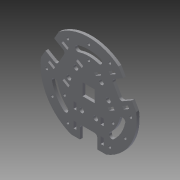
# Autodesk Inventor part: pcb
Saved by Autodesk Inventor 2015 (Build 190159000, 159)
## iProperties
Created: 2015-10-17
Part Number: pcb
Material: Polycarbonate, Clear
Document SubType Name: Modeling
Designer: Brian
Density: 1.2 g/cm^3
Appearance: Default
Mass: 22.2176 g
Surface Area: 156.183 cm^2
Volume: 18.5147 cm^3
Author: Brian
Autodesk Inventor part; units mm, degrees
ref_plane "YZ Plane" through (0, 0, 0) normal (1, 0, 0) x (0, 1, 0)
ref_plane "XZ Plane" through (0, 0, 0) normal (0, 1, 0) x (-1, 0, 0)
ref_plane "XY Plane" through (0, 0, 0) normal (0, 0, 1) x (1, 0, 0)
sketch "Sketch1" plane through (0, 0, 0) normal (0, 1, 0) x (-1, 0, 0)
  line L0 (0, 0) -> (0, -47.907) construction
  line L1 (0, -47.907) -> (18.8989, -47.907)
  line L2 (0, -47.907) -> (-18.8989, -47.907)
  line L3 (-41.4887, 23.9535) -> (0, 0) construction
  line L4 (0, 0) -> (41.4887, 23.9535) construction
  line L5 (41.4887, 23.9535) -> (32.0392, 40.3204)
  line L6 (-41.4887, 23.9535) -> (-50.9381, 7.5866)
  line L7 (-41.4887, 23.9535) -> (-32.0392, 40.3204)
  line L8 (41.4887, 23.9535) -> (50.9381, 7.5866)
  arc A0 (18.8989, -47.907) -> (50.9381, 7.5866) centre (0, 0) ccw
  arc A1 (32.0392, 40.3204) -> (-32.0392, 40.3204) centre (0, 0) ccw
  arc A2 (-50.9381, 7.5866) -> (-18.8989, -47.907) centre (0, 0) ccw
  dimension "d1" = 47.907
  dimension "d2" = 120
  dimension "d3" = 120
  dimension "d4" = 47.907
  dimension "d5" = 47.907
  dimension "d6" = 51.5
  dimension "d7" = 51.5
  dimension "d8" = 51.5
  constraints: 18 end point, 6 point on circle, 3 centre point, 3 perpendicular, 2 point on line, 1 coincident, 1 horizontal, 1 vertical
  measures "d1" distance of L0.start L0.end
  measures "d2" angle of L4 L0
  measures "d3" angle of L3 L4
  measures "d4" distance of L3.start L0.start
  measures "d5" distance of L0.start L4.end
  measures "d6" radius of A1
  measures "d7" radius of A2
  measures "d8" radius of A0
extrude "Extrusion1" add sketch "Sketch1" along normal blind 3
sketch "Sketch2" plane through (0, 3, 0) normal (0, 1, 0) x (1, 0, 0)
  circle A0 centre (-7.5, 20.006) radius 2.5
  circle A1 centre (7.5, 20.006) radius 2.5
  line L0 (-7.5, 20.006) -> (7.5, 20.006) construction
  point P0 (0, 0)
  point P1 (0, 20.006)
  dimension "d11" = 5
  dimension "d12" = 5
  dimension "d13" = 20.006
  dimension "d14" = 15
  constraints: 2 centre point, 2 end point, 1 horizontal, 1 horizontal alignment, 1 midpoint, 1 vertical alignment
  measures "d11" diameter of A0
  measures "d12" diameter of A1
  measures "d13" distance from line of point (0, 0) L0
  measures "d14" distance of L0.start L0.end
sketch "Sketch3" plane through (0, 3, 0) normal (0, 1, 0) x (1, 0, 0)
  line L0 (18.8989, 47.907) -> (-18.8989, 47.907) construction
  arc A0 (-18.8989, 47.907) -> (-50.9381, -7.5866) centre (0, 0) ccw construction
  line L1 (-50.9381, -7.5866) -> (-32.0392, -40.3204) construction
  arc A1 (-32.0392, -40.3204) -> (32.0392, -40.3204) centre (0, 0) ccw construction
  line L2 (32.0392, -40.3204) -> (50.9381, -7.5866) construction
  arc A2 (50.9381, -7.5866) -> (18.8989, 47.907) centre (0, 0) ccw construction
  line L3 (18.8989, 47.907) -> (-18.8989, 47.907)
  line L4 (18.8989, 47.907) -> (-18.8989, 47.907) projected
  line L5 (16, 40.907) -> (-16, 40.907) construction
  line L6 (16, 33.907) -> (-16, 33.907) construction
  line L7 (16, 22.907) -> (-16, 22.907) construction
  line L8 (16, 15.907) -> (-16, 15.907) construction
  line L9 (16, 15.907) -> (16, 40.907) construction
  line L10 (-16, 40.907) -> (-16, 15.907) construction
  line L11 (-16, 40.907) -> (-13, 40.907)
  line L12 (-13, 40.907) -> (-13, 33.907)
  line L13 (-13, 33.907) -> (-16, 33.907)
  line L14 (-16, 33.907) -> (-16, 40.907)
  line L15 (-16, 22.907) -> (-13, 22.907)
  line L16 (-13, 22.907) -> (-13, 15.907)
  line L17 (-13, 15.907) -> (-16, 15.907)
  line L18 (-16, 15.907) -> (-16, 22.907)
  line L19 (16, 15.907) -> (13, 15.907)
  line L20 (13, 15.907) -> (13, 22.907)
  line L21 (13, 22.907) -> (16, 22.907)
  line L22 (16, 22.907) -> (16, 15.907)
  line L23 (16, 33.907) -> (13, 33.907)
  line L24 (13, 33.907) -> (13, 40.907)
  line L25 (13, 40.907) -> (16, 40.907)
  line L26 (16, 40.907) -> (16, 33.907)
  point P0 (0, 15.907)
  dimension "d15" = 7
  dimension "d16" = 7
  dimension "d17" = 11
  dimension "d18" = 7
  dimension "d19" = 32
  dimension "d20" = 3
  dimension "d21" = 3
  constraints: 46 end point, 10 equal length, 10 point on line, 5 horizontal, 4 perpendicular, 1 midpoint, 1 vertical, 1 vertical alignment
  measures "d15" distance between parallel lines of L0 L5
  measures "d16" distance between parallel lines of L5 L6
  measures "d17" distance between parallel lines of L6 L7
  measures "d18" distance between parallel lines of L7 L8
  measures "d19" distance between parallel lines of L10 L9
  measures "d20" distance of L12.end L13.end
  measures "d21" distance of L24.end L25.end
extrude "Extrusion2" cut sketch "Sketch2" against normal blind 3
extrude "Extrusion3" cut sketch "Sketch3" against normal blind 3
sketch "Sketch4" plane through (0, 3, 0) normal (0, 1, 0) x (1, 0, 0)
  line L0 (-9.25, 33.907) -> (9.25, 33.907)
  line L1 (9.25, 33.907) -> (9.25, 47.907)
  line L2 (9.25, 47.907) -> (-9.25, 47.907)
  line L3 (-9.25, 47.907) -> (-9.25, 33.907)
  line L4 (18.8989, 47.907) -> (-18.8989, 47.907) projected
  point P0 (0, 0)
  point P1 (0, 33.907)
  dimension "d26" = 18.5
  dimension "d28" = 14
  constraints: 8 end point, 2 parallel, 1 horizontal, 1 midpoint, 1 perpendicular, 1 point on line, 1 vertical alignment
  measures "d26" distance of L0.start L0.end
  measures "d28" distance of L0.end L1.end
extrude "Extrusion4" cut sketch "Sketch4" against normal blind 3
sketch "Sketch5" plane through (0, 3, 0) normal (0, 1, 0) x (1, 0, 0)
  line L0 (-6.4, -6.4) -> (6.4, -6.4)
  line L1 (6.4, -6.4) -> (6.4, 6.4)
  line L2 (6.4, 6.4) -> (-6.4, 6.4)
  line L3 (-6.4, 6.4) -> (-6.4, -6.4)
  point P0 (0, 0)
  point P1 (0, 6.4)
  point P2 (-6.4, 0)
  dimension "d31" = 12.8
  dimension "d32" = 12.8
  constraints: 8 end point, 2 midpoint, 2 parallel, 1 horizontal, 1 horizontal alignment, 1 perpendicular, 1 vertical alignment
  measures "d31" distance of L0.end L1.end
  measures "d32" distance of L1.end L2.end
extrude "Extrusion5" cut sketch "Sketch5" against normal blind 3
pattern_circular "Circular Pattern1" count 3 over 360 about axis through (0, 0, 0) along (0, 1, 0) of "Extrusion4", "Extrusion2", "Extrusion3"
sketch "Sketch6" plane through (0, 3, 0) normal (0, 1, 0) x (1, 0, 0)
  line L0 (33.9893, -8.9428) -> (46.1137, -15.9428) construction
  line L1 (46.1137, -15.9428) -> (50.9381, -7.5866) construction
  arc A0 (50.9381, -7.5866) -> (18.8989, 47.907) centre (0, 0) ccw construction
  line L2 (18.8989, 47.907) -> (9.25, 47.907) construction
  line L3 (9.25, 47.907) -> (9.25, 33.907) construction
  line L4 (9.25, 33.907) -> (-9.25, 33.907) construction
  line L5 (-9.25, 33.907) -> (-9.25, 47.907) construction
  line L6 (-9.25, 47.907) -> (-18.8989, 47.907) construction
  arc A1 (-18.8989, 47.907) -> (-50.9381, -7.5866) centre (0, 0) ccw construction
  line L7 (-50.9381, -7.5866) -> (-46.1137, -15.9428) construction
  line L8 (-46.1137, -15.9428) -> (-33.9893, -8.9428) construction
  line L9 (-33.9893, -8.9428) -> (-24.7393, -24.9642) construction
  line L10 (-24.7393, -24.9642) -> (-36.8637, -31.9642) construction
  line L11 (-36.8637, -31.9642) -> (-32.0392, -40.3204) construction
  arc A2 (-32.0392, -40.3204) -> (32.0392, -40.3204) centre (0, 0) ccw construction
  line L12 (32.0392, -40.3204) -> (36.8637, -31.9642) construction
  line L13 (36.8637, -31.9642) -> (24.7393, -24.9642) construction
  line L14 (24.7393, -24.9642) -> (33.9893, -8.9428) construction
  line L15 (21.7759, 5.9029) -> (27.838, 2.4029) construction
  line L16 (27.838, 2.4029) -> (26.338, -0.1952) construction
  line L17 (26.338, -0.1952) -> (20.2759, 3.3048) construction
  line L18 (20.2759, 3.3048) -> (21.7759, 5.9029) construction
  line L19 (37.3643, -3.0971) -> (43.4265, -6.5971) construction
  line L20 (43.4265, -6.5971) -> (41.9265, -9.1952) construction
  line L21 (41.9265, -9.1952) -> (35.8643, -5.6952) construction
  line L22 (35.8643, -5.6952) -> (37.3643, -3.0971) construction
  line L23 (27.4265, -34.3099) -> (21.3643, -30.8099) construction
  line L24 (21.3643, -30.8099) -> (22.8643, -28.2118) construction
  line L25 (22.8643, -28.2118) -> (28.9265, -31.7118) construction
  line L26 (28.9265, -31.7118) -> (27.4265, -34.3099) construction
  line L27 (11.838, -25.3099) -> (5.7759, -21.8099) construction
  line L28 (5.7759, -21.8099) -> (7.2759, -19.2118) construction
  line L29 (7.2759, -19.2118) -> (13.338, -22.7118) construction
  line L30 (13.338, -22.7118) -> (11.838, -25.3099) construction
  circle A3 centre (21.0757, -3.5078) radius 2.5 construction
  circle A4 centre (13.5757, -16.4982) radius 2.5 construction
  line L31 (-5.7759, -21.8099) -> (-11.838, -25.3099) construction
  line L32 (-11.838, -25.3099) -> (-13.338, -22.7118) construction
  line L33 (-13.338, -22.7118) -> (-7.2759, -19.2118) construction
  line L34 (-7.2759, -19.2118) -> (-5.7759, -21.8099) construction
  line L35 (-21.3643, -30.8099) -> (-27.4265, -34.3099) construction
  line L36 (-27.4265, -34.3099) -> (-28.9265, -31.7118) construction
  line L37 (-28.9265, -31.7118) -> (-22.8643, -28.2118) construction
  line L38 (-22.8643, -28.2118) -> (-21.3643, -30.8099) construction
  line L39 (-43.4265, -6.5971) -> (-37.3643, -3.0971) construction
  line L40 (-37.3643, -3.0971) -> (-35.8643, -5.6952) construction
  line L41 (-35.8643, -5.6952) -> (-41.9265, -9.1952) construction
  line L42 (-41.9265, -9.1952) -> (-43.4265, -6.5971) construction
  line L43 (-27.838, 2.4029) -> (-21.7759, 5.9029) construction
  line L44 (-21.7759, 5.9029) -> (-20.2759, 3.3048) construction
  line L45 (-20.2759, 3.3048) -> (-26.338, -0.1952) construction
  line L46 (-26.338, -0.1952) -> (-27.838, 2.4029) construction
  circle A5 centre (-13.5757, -16.4982) radius 2.5 construction
  circle A6 centre (-21.0757, -3.5078) radius 2.5 construction
  line L47 (6.4, 6.4) -> (6.4, -6.4) construction
  line L48 (6.4, -6.4) -> (-6.4, -6.4) construction
  line L49 (-6.4, -6.4) -> (-6.4, 6.4) construction
  line L50 (-6.4, 6.4) -> (6.4, 6.4) construction
  line L51 (-16, 15.907) -> (-16, 22.907) construction
  line L52 (-16, 22.907) -> (-13, 22.907) construction
  line L53 (-13, 22.907) -> (-13, 15.907) construction
  line L54 (-13, 15.907) -> (-16, 15.907) construction
  line L55 (-16, 33.907) -> (-16, 40.907) construction
  line L56 (-16, 40.907) -> (-13, 40.907) construction
  line L57 (-13, 40.907) -> (-13, 33.907) construction
  line L58 (-13, 33.907) -> (-16, 33.907) construction
  line L59 (16, 40.907) -> (16, 33.907) construction
  line L60 (16, 33.907) -> (13, 33.907) construction
  line L61 (13, 33.907) -> (13, 40.907) construction
  line L62 (13, 40.907) -> (16, 40.907) construction
  line L63 (16, 22.907) -> (16, 15.907) construction
  line L64 (16, 15.907) -> (13, 15.907) construction
  line L65 (13, 15.907) -> (13, 22.907) construction
  line L66 (13, 22.907) -> (16, 22.907) construction
  circle A7 centre (-7.5, 20.006) radius 2.5 construction
  circle A8 centre (7.5, 20.006) radius 2.5 construction
  circle A9 centre (38.9711, 22.5) radius 1.5
  circle A10 centre (-38.9711, 22.5) radius 1.5
  circle A11 centre (0, -45) radius 1.5
  circle A12 centre (0, 0) radius 45 construction
  line L67 (0, 0) -> (38.9711, 22.5) construction
  line L68 (0, 0) -> (-38.9711, 22.5) construction
  circle A13 centre (0, 0) radius 30 construction
  circle A14 centre (25.9808, 15) radius 1.5
  circle A15 centre (-25.9808, 15) radius 1.5
  circle A16 centre (0, -30) radius 1.5
  circle A17 centre (-22.5, -38.9711) radius 1.5
  circle A18 centre (22.5, -38.9711) radius 1.5
  circle A19 centre (45, 0) radius 1.5
  circle A20 centre (22.5, 38.9711) radius 1.5
  circle A21 centre (-22.5, 38.9711) radius 1.5
  circle A22 centre (-45, 0) radius 1.5
  line L69 (0, 0) -> (-22.5, -38.9711) construction
  line L70 (0, 0) -> (22.5, -38.9711) construction
  line L71 (0, 0) -> (-22.5, 38.9711) construction
  line L72 (0, 0) -> (-45, 0) construction
  line L73 (45, 0) -> (0, 0) construction
  line L74 (22.5, 38.9711) -> (0, 0) construction
  line L75 (0, 0) -> (0, 33.907) construction
  line L76 (0, 0) -> (-29.3643, -16.9535) construction
  line L77 (-24.7393, -24.9642) -> (-33.9893, -8.9428) construction
  line L78 (0, 0) -> (29.3643, -16.9535) construction
  dimension "d43" = 90
  dimension "d38" = 3
  dimension "d39" = 3
  dimension "d40" = 3
  dimension "d41" = 120
  dimension "d42" = 120
  dimension "d44" = 60
  dimension "d45" = 3
  dimension "d46" = 3
  dimension "d47" = 3
  dimension "d63" = 3
  dimension "d64" = 3
  dimension "d65" = 3
  dimension "d66" = 3
  dimension "d67" = 30
  dimension "d68" = 30
  dimension "d69" = 30
  dimension "d70" = 30
  dimension "d71" = 30
  dimension "d72" = 30
  dimension "d73" = 3
  dimension "d74" = 3
  constraints: 22 end point, 13 centre point, 4 midpoint, 4 point on line, 3 coincident, 3 point on circle, 2 vertical alignment, 11 other
  measures "d38" diameter of A9
  measures "d39" diameter of A10
  measures "d40" diameter of A11
  measures "d41" angle of L47 L67
  measures "d42" angle of L68 L49
  measures "d44" diameter of A13
  measures "d45" diameter of A14
  measures "d46" diameter of A15
  measures "d47" diameter of A16
  measures "d63" diameter of A22
  measures "d64" diameter of A21
  measures "d65" diameter of A18
  measures "d66" diameter of A17
  measures "d67" angle of L71 L75
  measures "d68" angle of L74 L75
  measures "d69" angle of L76 L69
  measures "d70" angle of L72 L76
  measures "d71" angle of L78 L73
  measures "d72" angle of L78 L70
  measures "d73" diameter of A19
  measures "d74" diameter of A20
extrude "Extrusion6" cut sketch "Sketch6" against normal blind 3
sketch "Sketch7" plane through (0, 0, 0) normal (0, -1, 0) x (1, 0, 0)
  circle A0 centre (-25.9808, -15) radius 1.5 construction
  circle A1 centre (0, 45) radius 1.5 construction
  circle A2 centre (38.9711, -22.5) radius 1.5 construction
  circle A3 centre (-38.9711, -22.5) radius 1.5 construction
  circle A4 centre (25.9808, -15) radius 1.5 construction
  circle A5 centre (0, 30) radius 1.5 construction
  line L0 (-16, -22.907) -> (-16, -15.907) construction
  line L1 (-16, -15.907) -> (-13, -15.907) construction
  line L2 (-13, -15.907) -> (-13, -22.907) construction
  line L3 (-13, -22.907) -> (-16, -22.907) construction
  line L4 (-16, -40.907) -> (-16, -33.907) construction
  line L5 (-16, -33.907) -> (-13, -33.907) construction
  line L6 (-13, -33.907) -> (-13, -40.907) construction
  line L7 (-13, -40.907) -> (-16, -40.907) construction
  line L8 (16, -33.907) -> (16, -40.907) construction
  line L9 (16, -40.907) -> (13, -40.907) construction
  line L10 (13, -40.907) -> (13, -33.907) construction
  line L11 (13, -33.907) -> (16, -33.907) construction
  line L12 (16, -15.907) -> (16, -22.907) construction
  line L13 (16, -22.907) -> (13, -22.907) construction
  line L14 (13, -22.907) -> (13, -15.907) construction
  line L15 (13, -15.907) -> (16, -15.907) construction
  circle A6 centre (-7.5, -20.006) radius 2.5 construction
  circle A7 centre (7.5, -20.006) radius 2.5 construction
  line L16 (46.1137, 15.9428) -> (33.9893, 8.9428) construction
  line L17 (33.9893, 8.9428) -> (24.7393, 24.9642) construction
  line L18 (24.7393, 24.9642) -> (36.8637, 31.9642) construction
  line L19 (32.0392, 40.3204) -> (36.8637, 31.9642) construction
  arc A8 (32.0392, 40.3204) -> (-32.0392, 40.3204) centre (0, 0) ccw construction
  line L20 (-36.8637, 31.9642) -> (-32.0392, 40.3204) construction
  line L21 (-36.8637, 31.9642) -> (-24.7393, 24.9642) construction
  line L22 (-24.7393, 24.9642) -> (-33.9893, 8.9428) construction
  line L23 (-33.9893, 8.9428) -> (-46.1137, 15.9428) construction
  line L24 (-50.9381, 7.5866) -> (-46.1137, 15.9428) construction
  arc A9 (-50.9381, 7.5866) -> (-18.8989, -47.907) centre (0, 0) ccw construction
  line L25 (-9.25, -47.907) -> (-18.8989, -47.907) construction
  line L26 (-9.25, -47.907) -> (-9.25, -33.907) construction
  line L27 (-9.25, -33.907) -> (9.25, -33.907) construction
  line L28 (9.25, -33.907) -> (9.25, -47.907) construction
  line L29 (18.8989, -47.907) -> (9.25, -47.907) construction
  arc A10 (18.8989, -47.907) -> (50.9381, 7.5866) centre (0, 0) ccw construction
  line L30 (46.1137, 15.9428) -> (50.9381, 7.5866) construction
  line L31 (6.4, 6.4) -> (6.4, -6.4) construction
  line L32 (6.4, -6.4) -> (-6.4, -6.4) construction
  line L33 (-6.4, -6.4) -> (-6.4, 6.4) construction
  line L34 (-6.4, 6.4) -> (6.4, 6.4) construction
  circle A11 centre (-21.0757, 3.5078) radius 2.5 construction
  circle A12 centre (-13.5757, 16.4982) radius 2.5 construction
  line L35 (-21.7759, -5.9029) -> (-27.838, -2.4029) construction
  line L36 (-27.838, -2.4029) -> (-26.338, 0.1952) construction
  line L37 (-26.338, 0.1952) -> (-20.2759, -3.3048) construction
  line L38 (-20.2759, -3.3048) -> (-21.7759, -5.9029) construction
  line L39 (-37.3643, 3.0971) -> (-43.4265, 6.5971) construction
  line L40 (-43.4265, 6.5971) -> (-41.9265, 9.1952) construction
  line L41 (-41.9265, 9.1952) -> (-35.8643, 5.6952) construction
  line L42 (-35.8643, 5.6952) -> (-37.3643, 3.0971) construction
  line L43 (-27.4265, 34.3099) -> (-21.3643, 30.8099) construction
  line L44 (-21.3643, 30.8099) -> (-22.8643, 28.2118) construction
  line L45 (-22.8643, 28.2118) -> (-28.9265, 31.7118) construction
  line L46 (-28.9265, 31.7118) -> (-27.4265, 34.3099) construction
  line L47 (-11.838, 25.3099) -> (-5.7759, 21.8099) construction
  line L48 (-5.7759, 21.8099) -> (-7.2759, 19.2118) construction
  line L49 (-7.2759, 19.2118) -> (-13.338, 22.7118) construction
  line L50 (-13.338, 22.7118) -> (-11.838, 25.3099) construction
  circle A13 centre (13.5757, 16.4982) radius 2.5 construction
  circle A14 centre (21.0757, 3.5078) radius 2.5 construction
  line L51 (5.7759, 21.8099) -> (11.838, 25.3099) construction
  line L52 (11.838, 25.3099) -> (13.338, 22.7118) construction
  line L53 (13.338, 22.7118) -> (7.2759, 19.2118) construction
  line L54 (7.2759, 19.2118) -> (5.7759, 21.8099) construction
  line L55 (21.3643, 30.8099) -> (27.4265, 34.3099) construction
  line L56 (27.4265, 34.3099) -> (28.9265, 31.7118) construction
  line L57 (28.9265, 31.7118) -> (22.8643, 28.2118) construction
  line L58 (22.8643, 28.2118) -> (21.3643, 30.8099) construction
  line L59 (43.4265, 6.5971) -> (37.3643, 3.0971) construction
  line L60 (37.3643, 3.0971) -> (35.8643, 5.6952) construction
  line L61 (35.8643, 5.6952) -> (41.9265, 9.1952) construction
  line L62 (41.9265, 9.1952) -> (43.4265, 6.5971) construction
  line L63 (27.838, -2.4029) -> (21.7759, -5.9029) construction
  line L64 (21.7759, -5.9029) -> (20.2759, -3.3048) construction
  line L65 (20.2759, -3.3048) -> (26.338, 0.1952) construction
  line L66 (26.338, 0.1952) -> (27.838, -2.4029) construction
  arc A15 (-39.1259, -8.3165) -> (-26.7652, -29.7258) centre (0, 0) ccw
  arc A16 (-33.257, -7.069) -> (-22.7504, -25.2669) centre (0, 0) ccw
  arc A17 (-33.257, -7.069) -> (-39.1259, -8.3165) centre (-36.1915, -7.6927) ccw
  arc A18 (-26.7652, -29.7258) -> (-22.7504, -25.2669) centre (-24.7578, -27.4964) ccw
  line L67 (-36.1915, -7.6927) -> (0, 0) construction
  line L68 (0, 0) -> (-24.7578, -27.4964) construction
  line L69 (0, 0) -> (0, -33.907) construction
  line L70 (0, 0) -> (-29.3643, 16.9535) construction
  line L71 (-24.7393, 24.9642) -> (-33.9893, 8.9428) construction
  dimension "d50" = 42
  dimension "d51" = 42
  dimension "d52" = 6
  dimension "d53" = 34
  constraints: 8 end point, 8 point on circle, 4 centre point, 4 tangent, 2 coincident, 2 midpoint
  measures "d50" angle of L70 L67
  measures "d51" angle of L69 L68
  measures "d52" radial gap between concentric circles of A16 A15
  measures "d53" radius of A16
extrude "Extrusion7" cut sketch "Sketch7" against normal blind 3
pattern_circular "Circular Pattern2" count 3 over 360 about axis through (0, 0, 0) along (0, 1, 0) of "Extrusion7"
fillet "Fillet1" radius 3 2 edges at (9.25, 1.5, -33.907) (-9.25, 1.5, -33.907)
pattern_circular "Circular Pattern3" count 3 over 360 about axis through (0, 0, 0) along (0, 1, 0) of "Fillet1"
equation "\"d4\" = d1"
equation "\"d5\" = d1"
equation "\"d6\" = d8"
equation "\"d7\" = d8"
equation "\"d12\" = d11"
equation "\"d21\" = d20"
equation "\"d32\" = d31"
equation "\"d39\" = d38"
equation "\"d40\" = d38"
equation "\"d45\" = d38"
equation "\"d46\" = d38"
equation "\"d47\" = d38"
equation "\"d63\" = d38"
equation "\"d64\" = d38"
equation "\"d65\" = d38"
equation "\"d66\" = d38"
equation "\"d68\" = d67"
equation "\"d69\" = d67"
equation "\"d70\" = d67"
equation "\"d71\" = d67"
equation "\"d72\" = d67"
equation "\"d73\" = d38"
equation "\"d74\" = d38"
equation "\"d51\" = d50"
body "Solid1"
